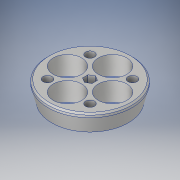
# Autodesk Inventor part: Flywheel Half
Saved by Autodesk Inventor 2019.4 (Build 234330000, 330)
## iProperties
Created: 2020-01-16
Part Number: Flywheel Half
Material: Aluminum 6061
Document SubType Name: Modeling
Designer: admin
Density: 2.7 g/cm^3
Appearance: Aluminum - Flat
Mass: 277.559 g
Surface Area: 319.263 cm^2
Volume: 102.8 cm^3
Author: admin
Autodesk Inventor part; units mm, degrees
ref_plane "YZ Plane" through (0, 0, 0) normal (1, 0, 0) x (0, 1, 0)
ref_plane "XZ Plane" through (0, 0, 0) normal (0, 1, 0) x (-1, 0, 0)
ref_plane "XY Plane" through (0, 0, 0) normal (0, 0, 1) x (1, 0, 0)
sketch "Sketch1" plane through (0, 0, 0) normal (1, 0, 0) x (0, 1, 0)
  line L0 (12.5, 55.88) -> (7.5, 55.88)
  line L1 (-12.5, 55.88) -> (-12.5, 50.88) construction
  line L2 (-12.5, 0) -> (12.5, 0)
  line L3 (12.5, 0) -> (12.5, 55.88)
  line L4 (7.5, 55.88) -> (-12.5, 50.88)
  line L5 (7.5, 55.88) -> (-12.5, 55.88) construction
  line L6 (-12.5, 50.88) -> (-12.5, 0)
  point P0 (0, 0)
  point P1 (0, 0)
  dimension "d0" = 55.88
  dimension "d1" = 25
  dimension "d2" = 5
  dimension "d3" = 20
  constraints: 14 end point, 4 parallel, 4 perpendicular, 2 horizontal, 1 coincident, 1 midpoint
  measures "d0" distance of L2.end L0.start
  measures "d1" distance of L0.start L1.start
  measures "d2" vertical distance of L0.end L1.end
  measures "d3" horizontal distance of L0.end L1.end
revolve "Revolution1" add sketch "Sketch1" angle 360 about axis through (0, -12.5, 0) along (0, 1, 0)
chamfer "Chamfer1" distance 2 angle 45 1 edges at (0, 12.5, -55.88)
sketch "Sketch2" plane through (0, -12.5, 0) normal (0, -1, 0) x (1, 0, 0)
  line L0 (-6.35, 3.6662) -> (0, 7.3323)
  line L1 (0, 7.3323) -> (6.35, 3.6662)
  line L2 (6.35, 3.6662) -> (6.35, -3.6662)
  line L3 (6.35, -3.6662) -> (0, -7.3323)
  line L4 (0, -7.3323) -> (-6.35, -3.6662)
  line L5 (-6.35, -3.6662) -> (-6.35, 3.6662)
  circle A0 centre (30, 0) radius 19
  line L6 (30, 0) -> (0, 0) construction
  circle A1 centre (28.2843, -28.2843) radius 6
  line L7 (0, 0) -> (28.2843, -28.2843) construction
  circle A2 centre (0, 30) radius 19
  circle A3 centre (28.2843, 28.2843) radius 6
  circle A4 centre (-30, 0) radius 19
  circle A5 centre (-28.2843, 28.2843) radius 6
  circle A6 centre (0, -30) radius 19
  circle A7 centre (-28.2843, -28.2843) radius 6
  dimension "d8" = 12.7
  dimension "d9" = 38
  dimension "d10" = 30
  dimension "d11" = 12
  dimension "d12" = 45
  dimension "d13" = 40
  dimension "d16" = 360
  constraints: 16 end point, 8 centre point, 1 coincident, 1 horizontal, 1 vertical, 30 other
  measures "d8" distance between parallel lines of L2 L5
  measures "d9" diameter of A0
  measures "d10" distance of L6.start L6.end
  measures "d11" diameter of A1
  measures "d12" angle of L6 L7
  measures "d13" distance of L6.end L7.end
extrude "Extrusion1" cut sketch "Sketch2" against normal through all
body "Solid1"
